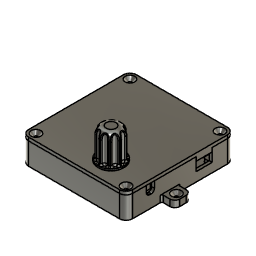
case_esp32_switch_v12 (Autodesk Fusion 360 design; units mm, degrees)
Autodesk Fusion 360 part; units mm, degrees
sketch "Skizze1" plane through (0, 0, 0) normal (0, 0, 1) x (1, 0, 0)
  line L0 (-30, 17.5) -> (30, 17.5)
  line L1 (30, 17.5) -> (30, -17.5)
  line L2 (30, -17.5) -> (-30, -17.5)
  line L3 (-30, -17.5) -> (-30, 17.5)
  line L4 (27.5, -15) -> (-27.5, -15) construction
  line L5 (-27.5, -15) -> (-27.5, 15) construction
  line L6 (-27.5, 15) -> (27.5, 15) construction
  line L7 (27.5, 15) -> (27.5, -15) construction
  line L8 (-22.2, 17.5) -> (-4.2, 17.5)
  line L9 (-4.2, 17.5) -> (-4.2, 22.9)
  line L10 (-4.2, 22.9) -> (-22.2, 22.9)
  line L11 (-22.2, 22.9) -> (-22.2, 17.5)
  line L12 (-30, 1.6) -> (-24, 1.6)
  line L13 (-24, 1.6) -> (-24, -7.6)
  line L14 (-24, -7.6) -> (-30, -7.6)
  line L15 (-30, -7.6) -> (-30, 1.6)
  line L16 (30, 11.5) -> (21, 11.5)
  line L17 (21, 11.5) -> (21, 1.6)
  line L18 (21, 1.6) -> (30, 1.6)
  line L19 (30, 1.6) -> (30, 11.5)
  line L20 (0, 17.5) -> (0, 0) construction
  line L21 (0, 0) -> (-30, 0) construction
  line L22 (30.2, -17.7) -> (-30.2, -17.7)
  line L23 (-30.2, -17.7) -> (-30.2, 17.7)
  line L24 (-30.2, 17.7) -> (30.2, 17.7)
  line L25 (30.2, 17.7) -> (30.2, -17.7)
  line L26 (-32, -41.5) -> (-32, 24.9)
  line L27 (-32, 24.9) -> (32, 24.9)
  line L28 (32, 24.9) -> (32, -41.5)
  line L29 (32, -41.5) -> (-32, -41.5)
  line L30 (-30.2, 17.7) -> (-30.2, 23.1)
  line L31 (-30.2, 23.1) -> (32, 23.1)
  line L32 (-30, 1.6) -> (-32, 1.6)
  line L33 (-30, -7.6) -> (-32, -7.6)
  line L34 (30, 11.5) -> (32, 11.5)
  line L35 (30, 1.6) -> (32, 1.6)
  line L36 (25.2, 17.7) -> (30.2, 17.7)
  line L37 (30.2, 17.7) -> (30.2, 12.7)
  line L38 (30.2, 12.7) -> (25.2, 12.7)
  line L39 (25.2, 12.7) -> (25.2, 17.7)
  line L40 (-30.2, 17.7) -> (-25.2, 17.7)
  line L41 (-25.2, 17.7) -> (-25.2, 12.7)
  line L42 (-25.2, 12.7) -> (-30.2, 12.7)
  line L43 (-30.2, 12.7) -> (-30.2, 17.7)
  line L44 (-30.2, -17.7) -> (-25.2, -17.7)
  line L45 (-25.2, -17.7) -> (-25.2, -12.7)
  line L46 (-25.2, -12.7) -> (-30.2, -12.7)
  line L47 (-30.2, -12.7) -> (-30.2, -17.7)
  line L48 (30.2, -17.7) -> (25.2, -17.7)
  line L49 (25.2, -17.7) -> (25.2, -12.7)
  line L50 (25.2, -12.7) -> (30.2, -12.7)
  line L51 (30.2, -12.7) -> (30.2, -17.7)
  line L52 (30.2, -17.7) -> (30.2, -39.7)
  line L53 (30.2, -39.7) -> (-30.2, -39.7)
  line L54 (-30.2, -39.7) -> (-30.2, -17.7)
  line L55 (-4.3, -19.2) -> (22.2, -19.2)
  line L56 (22.2, -19.2) -> (22.2, -38)
  line L57 (22.2, -38) -> (-4.3, -38)
  line L58 (-4.3, -38) -> (-4.3, -19.2)
  line L59 (22.2, -21.45) -> (-4.3, -21.45) construction
  line L60 (30.2, 17.7) -> (30.2, 23.1)
  line L61 (22.2, -23.3) -> (-4.3, -23.3)
  line L62 (22.2, -36) -> (-4.3, -36)
  line L63 (-30.2, 23.1) -> (-25.2, 23.1)
  line L64 (-25.2, 23.1) -> (-25.2, 18.1)
  line L65 (-25.2, 18.1) -> (-30.2, 18.1)
  line L66 (-30.2, 18.1) -> (-30.2, 23.1)
  line L67 (30.2, 23.1) -> (25.2, 23.1)
  line L68 (25.2, 23.1) -> (25.2, 18.1)
  line L69 (25.2, 18.1) -> (30.2, 18.1)
  line L70 (30.2, 18.1) -> (30.2, 23.1)
  line L71 (30.2, -39.7) -> (25.2, -39.7)
  line L72 (25.2, -39.7) -> (25.2, -34.7)
  line L73 (25.2, -34.7) -> (30.2, -34.7)
  line L74 (30.2, -34.7) -> (30.2, -39.7)
  line L75 (-30.2, -39.7) -> (-25.2, -39.7)
  line L76 (-25.2, -39.7) -> (-25.2, -34.7)
  line L77 (-25.2, -34.7) -> (-30.2, -34.7)
  line L78 (-30.2, -34.7) -> (-30.2, -39.7)
  line L79 (23.4, -39.2) -> (-5.5, -39.2)
  line L80 (-5.5, -39.2) -> (-5.5, -18)
  line L81 (-5.5, -18) -> (23.4, -18)
  line L82 (23.4, -18) -> (23.4, -39.2)
  line L83 (-4.3, -23.3) -> (-5.5, -23.3)
  line L84 (22.2, -23.3) -> (23.4, -23.3)
  line L85 (22.2, -36) -> (23.4, -36)
  line L86 (-4.3, -36) -> (-5.5, -36)
  point P0 (2.7, -21.45)
  point P1 (16.4, -21.45)
  dimension "d1" = 35
  dimension "d2" = 60
  dimension "d3" = 2.5
  dimension "d4" = 18
  dimension "d5" = 7.8
  dimension "d6" = 9.2
  dimension "d7" = 9.9
  dimension "d8" = 5.4
  dimension "d9" = 9.9
  dimension "d10" = 6
  dimension "d11" = 9
  dimension "d12" = 6
  dimension "d13" = -0.2
  dimension "d14" = 2
  dimension "d15" = 1.8
  dimension "d16" = 1.8
  dimension "d17" = 1.8
  dimension "d18" = 5
  dimension "d19" = 5
  dimension "d20" = 5
  dimension "d21" = 5
  dimension "d22" = 22
  dimension "d23" = 1.8
  dimension "d24" = 26.5
  dimension "d25" = 18.8
  dimension "d26" = 8
  dimension "d27" = 2.25
  dimension "d28" = 13.7
  dimension "d29" = 7
  dimension "d30" = 1.5
  dimension "d38" = 4.1
  dimension "d39" = 2
  dimension "d43" = 5
  dimension "d44" = 5
  dimension "d45" = 5
  dimension "d46" = 5
  dimension "d57" = -1.2
  constraint horizontal L0
  constraint vertical L1
  constraint horizontal L2
  constraint vertical L3
  constraint horizontal L8
  constraint vertical L9
  constraint horizontal L10
  constraint vertical L11
  constraint coincident L0 L8.start
  constraint horizontal L12
  constraint vertical L13
  constraint horizontal L14
  constraint vertical L15
  constraint coincident L3 L12.start
  constraint horizontal L16
  constraint vertical L17
  constraint horizontal L18
  constraint vertical L19
  constraint coincident L1 L16.start
  constraint midpoint L0 L20.start
  constraint coincident L20.end L21.start
  constraint midpoint L3 L21.end
  constraint horizontal L21
  constraint vertical L20
  constraint vertical L26
  constraint perpendicular L26 L27
  constraint perpendicular L27 L28
  constraint perpendicular L26 L29
  constraint perpendicular L27 L30
  constraint coincident L28 L31.end
  constraint perpendicular L28 L31
  constraint coincident L26 L32.end
  constraint perpendicular L26 L32
  constraint coincident L26 L33.end
  constraint perpendicular L26 L33
  constraint coincident L28 L34.end
  constraint perpendicular L28 L34
  constraint coincident L28 L35.end
  constraint perpendicular L28 L35
  constraint horizontal L36
  constraint vertical L37
  constraint horizontal L38
  constraint vertical L39
  constraint coincident L25 L37.end
  constraint coincident L24 L36.start
  constraint horizontal L40
  constraint vertical L41
  constraint horizontal L42
  constraint vertical L43
  constraint horizontal L44
  constraint vertical L45
  constraint horizontal L46
  constraint vertical L47
  constraint horizontal L48
  constraint vertical L49
  constraint horizontal L50
  constraint vertical L51
  constraint collinear L39 L49
  constraint collinear L46 L50
  constraint collinear L41 L45
  constraint collinear L38 L42
  constraint perpendicular L48 L52
  constraint perpendicular L25 L53
  constraint perpendicular L53 L54
  constraint horizontal L55
  constraint vertical L56
  constraint horizontal L57
  constraint vertical L58
  constraint coincident L56 L59.start
  constraint coincident L58 L59.end
  constraint perpendicular L58 L59
  constraint coincident L59 P0
  constraint coincident L59 P1
  constraint perpendicular L31 L60
  constraint coincident L56 L61.start
  constraint coincident L58 L61.end
  constraint perpendicular L58 L61
  constraint coincident L56 L62.start
  constraint coincident L58 L62.end
  constraint perpendicular L58 L62
  constraint horizontal L63
  constraint vertical L64
  constraint horizontal L65
  constraint vertical L66
  constraint horizontal L67
  constraint vertical L68
  constraint horizontal L69
  constraint vertical L70
  constraint horizontal L71
  constraint vertical L72
  constraint horizontal L73
  constraint vertical L74
  constraint horizontal L75
  constraint vertical L76
  constraint horizontal L77
  constraint vertical L78
  constraint collinear L64 L76
  constraint collinear L73 L77
  constraint collinear L68 L72
  constraint collinear L65 L69
  constraint coincident L80 L83.end
  constraint perpendicular L80 L83
  constraint coincident L82 L84.end
  constraint perpendicular L82 L84
  constraint coincident L82 L85.end
  constraint perpendicular L82 L85
  constraint coincident L80 L86.end
  constraint perpendicular L80 L86
  measures "d1" distance of L0 L2
  measures "d2" distance of L1 L3
  measures "d4" distance of L9.end L10.end
  measures "d5" distance of L3 L11
  measures "d6" distance of L12.end L13.end
  measures "d7" distance of L2 L14
  measures "d8" distance of L8.start L10.end
  measures "d9" distance of L16.end L17.end
  measures "d10" distance of L0 L16
  measures "d11" distance of L17.end L18.end
  measures "d12" distance of L13.end L14.end
  measures "d14" distance of L10 L27
  measures "d15" distance of L26 L30
  measures "d16" distance of L27 L31
  measures "d17" distance of L25 L28
  measures "d18" distance of L37 L39
  measures "d19" distance of L24 L38
  measures "d20" distance of L45.end L46.end
  measures "d21" distance of L44.end L45.end
  measures "d22" distance of L22 L53
  measures "d23" distance of L29 L53
  measures "d24" distance of L56.end L57.end
  measures "d25" distance of L55.end L56.end
  measures "d26" distance of L52 L56
  measures "d27" distance of L55 L59
  measures "d28" distance of P0 P1
  measures "d29" distance of L58 P0
  measures "d30" distance of L22 L55
  measures "d38" distance of L55 L61
  measures "d39" distance of L57 L62
  measures "d43" distance of L64.end L65.end
  measures "d44" distance of L63.end L64.end
  measures "d45" distance of L75.end L76.end
  measures "d46" distance of L60 L68
extrude "Extrusion1" add sketch "Skizze1" against normal blind 2 contours L0 L8 L9 L11 L24 | L0 L1 L2 L3 L8 L12 L13 L14 L16 L17 L18 L38 L39 L41 L42 L45 L46 L49 L50 | L0 L11 L24 L41 | L0 L9 L24 L39 | L0 L3 L41 L42 | L0 L3 L23 L24 L40 L41 L42 L43 | L9 L10 L11 L24 L30 L31 L36 L40 L60 L64 L65 L68 L69 | L9 L10 L11 L24 | L0 L1 L24 L25 L36 L37 L38 L39 | L0 L1 L38 L39 | L3 L23 L32 L42 | L23 L26 L27 L28 L30 L31 L32 L43 L63 L66 L67 | L1 L25 L34 L38 | L25 L28 L31 L34 L37 L60 L70 | L3 L12 L13 L14 L15 | L3 L15 L23 L32 L33 | L30 L31 L63 L64 L65 L66 | L1 L19 L25 L34 L35 | L1 L16 L17 L18 L19 | L31 L60 L67 L68 L69 L70 | L3 L23 L33 L46 | L23 L26 L32 L33 | L1 L25 L35 L50 | L25 L28 L34 L35 | L2 L3 L45 L46 | L2 L3 L22 L23 L44 L45 L46 L47 | L23 L25 L26 L28 L29 L33 L35 L47 L51 L52 L53 L54 L71 L74 L75 L78 | L1 L2 L22 L25 L48 L49 L50 L51 | L1 L2 L49 L50 | L2 L22 L45 L49 | L22 L44 L48 L52 L53 L54 L72 L73 L76 L77 | L53 L54 L75 L76 L77 L78 | L52 L53 L71 L72 L73 L74 | L55 L56 L58 L80 L81 L82 L83 L84 | L55 L56 L58 L61 | L56 L58 L61 L62 | L58 L80 L83 L86 | L56 L82 L84 L85 | L56 L57 L58 L62 | L56 L57 L58 L79 L80 L82 L85 L86 makes body 1
extrude "Extrusion2" add sketch "Skizze1" along normal blind 2 contours L0 L3 L41 L42 | L0 L3 L23 L24 L40 L41 L42 L43 | L0 L1 L24 L25 L36 L37 L38 L39 | L0 L1 L38 L39 | L23 L26 L27 L28 L30 L31 L32 L43 L63 L66 L67 | L25 L28 L31 L34 L37 L60 L70 | L23 L26 L32 L33 | L25 L28 L34 L35 | L2 L3 L45 L46 | L2 L3 L22 L23 L44 L45 L46 L47 | L23 L25 L26 L28 L29 L33 L35 L47 L51 L52 L53 L54 L71 L74 L75 L78 | L1 L2 L22 L25 L48 L49 L50 L51 | L1 L2 L49 L50 | L55 L56 L58 L61 | L56 L57 L58 L62 bodies 1
extrude "Extrusion3" add sketch "Skizze1" along normal blind 1.55 from surface at 2 contours L23 L26 L27 L28 L30 L31 L32 L43 L63 L66 L67 | L25 L28 L31 L34 L37 L60 L70 | L23 L26 L32 L33 | L25 L28 L34 L35 | L23 L25 L26 L28 L29 L33 L35 L47 L51 L52 L53 L54 L71 L74 L75 L78 bodies 1
extrude "Extrusion4" add sketch "Skizze1" along normal blind 7.95 from surface at 3.55 contours L23 L26 L27 L28 L30 L31 L32 L43 L63 L66 L67 | L25 L28 L31 L34 L37 L60 L70 | L23 L25 L26 L28 L29 L33 L35 L47 L51 L52 L53 L54 L71 L74 L75 L78 bodies 1
extrude "Extrusion5" add sketch "Skizze1" along normal up to surface (10.5 mm away) contours L30 L31 L63 L64 L65 L66 | L31 L60 L67 L68 L69 L70 | L53 L54 L75 L76 L77 L78 | L52 L53 L71 L72 L73 L74 bodies 1
fillet "Abrundung1" radius 4 8 edges at (-32, -41.5, 4.75) (32, -41.5, 4.75) (-32, 24.9, 4.75) (32, 24.9, 4.75) (30.2, 23.1, 11) (-30.2, 23.1, 11) (-30.2, -39.7, 11) (30.2, -39.7, 11) on bodies 1
sketch "Skizze2" plane through (0, 0, 2) normal (0, 0, 1) x (-1, 0, 0)
  line L0 (-22.2, 23.3) -> (-22.2, 19.2)
  line L1 (-22.2, 19.2) -> (4.3, 19.2)
  line L2 (4.3, 19.2) -> (4.3, 23.3)
  line L3 (4.3, 23.3) -> (-22.2, 23.3)
  point P0 (-2.7, 21.45)
  point P1 (-2.7, 21.45)
  point P2 (-16.4, 21.45)
  point P3 (-16.4, 21.45)
  constraint coincident P1 P0
  constraint coincident P3 P2
sketch "Skizze3" plane through (0, 0, 2) normal (0, 0, 1) x (-1, 0, 0)
  line L0 (30.2, -17.7) -> (30.2, -12.7)
  line L1 (30.2, -12.7) -> (25.2, -12.7)
  line L2 (25.2, -12.7) -> (25.2, -17.7)
  line L3 (25.2, -17.7) -> (30.2, -17.7)
  point P0 (27.5, -15)
  point P1 (27.5, -15)
  point P2 (27.5, 15)
  point P3 (27.5, 15)
  point P4 (-27.5, 15)
  point P5 (-27.5, 15)
  point P6 (-27.5, -15)
  point P7 (-27.5, -15)
  constraint coincident P1 P0
  constraint coincident P3 P2
  constraint coincident P5 P4
  constraint coincident P7 P6
hole "Bohrung1" at (-27.5, -15, 2) at (-27.5, 15, 2) at (27.5, 15, 2) at (27.5, -15, 2) direction (0, 0, -1) diameter 1.4 depth 3 tip angle 180 bodies 1
hole "Bohrung2" at (2.7, -21.45, 2) at (16.4, -21.45, 2) direction (0, 0, -1) diameter 1.4 depth 3 tip angle 180 bodies 1
sketch "Skizze4" plane through (0, 0, 10.5) normal (0, 0, 1) x (-1, 0, 0)
  arc A0 (30.2, 35.7) -> (26.2, 39.7) centre (26.2, 35.7) ccw
  line L0 (26.2, 39.7) -> (25.2, 39.7)
  line L1 (25.2, 39.7) -> (25.2, 34.7)
  line L2 (25.2, 34.7) -> (30.2, 34.7)
  line L3 (30.2, 34.7) -> (30.2, 35.7)
extrude "Extrusion6" add sketch "Skizze1" along normal up to surface (4 mm away) contours L55 L56 L58 L80 L81 L82 L83 L84 | L56 L57 L58 L79 L80 L82 L85 L86 bodies 1
sketch "Skizze5" plane through (0, 0, 10.5) normal (0, 0, 1) x (-1, 0, 0)
  point P0 (27.7, 37.2)
  point P1 (27.7, -20.6)
  point P2 (-27.7, -20.6)
  point P3 (-27.7, 37.2)
hole "Bohrung3" at (-27.7, 20.6, 10.5) at (27.7, 20.6, 10.5) at (27.7, -37.2, 10.5) at (-27.7, -37.2, 10.5) direction (0, 0, -1) diameter 1.4 depth 8 tip angle 180 bodies 1
fillet "Abrundung2" radius 1.5 2 edges at (-31.1, 1.6, 3.55) (-31.1, -7.6, 3.55) on bodies 1
fillet "Abrundung3" radius 2 4 edges at (-25.2, -34.7, 5.25) (-25.2, 18.1, 5.25) (25.2, 18.1, 5.25) (25.2, -34.7, 5.25) on bodies 1
fillet "Abrundung4" radius 1 14 edges at (-25.2, -17.7, 1) (-25.2, -12.7, 1) (-25.2, 12.7, 1) (-25.2, 17.7, 1) (25.2, 12.7, 1) (25.2, 17.7, 1) (25.2, -12.7, 1) (25.2, -17.7, 1) (30.2, -17.7, 1) (30.2, -12.7, 1) (30.2, 12.7, 1) (-30.2, 12.7, 1) (-30.2, -17.7, 1) (-30.2, -12.7, 1) on bodies 1
sketch "Skizze6" plane through (0, 0, -2) normal (0, 0, -1) x (1, 0, 0)
  arc A0 (28, -24.9) -> (32, -20.9) centre (28, -20.9) ccw
  line L0 (32, -20.9) -> (32, 37.5)
  arc A1 (32, 37.5) -> (28, 41.5) centre (28, 37.5) ccw
  line L1 (28, 41.5) -> (-28, 41.5)
  arc A2 (-28, 41.5) -> (-32, 37.5) centre (-28, 37.5) ccw
  line L2 (-32, 37.5) -> (-32, -20.9)
  arc A3 (-32, -20.9) -> (-28, -24.9) centre (-28, -20.9) ccw
  line L3 (-28, -24.9) -> (28, -24.9)
  line L4 (-32, 9.5) -> (-40, 9.5)
  line L5 (-40, 9.5) -> (-40, 19.5)
  line L6 (-40, 19.5) -> (-32, 19.5)
  line L7 (-32, 19.5) -> (-32, 9.5)
  line L8 (32, 9.5) -> (40, 9.5)
  line L9 (40, 9.5) -> (40, 19.5)
  line L10 (40, 19.5) -> (32, 19.5)
  line L11 (32, 19.5) -> (32, 9.5)
  line L12 (32, 41.5) -> (-32, 41.5)
  dimension "d69" = 10
  dimension "d70" = 8
  dimension "d71" = 8
  dimension "d72" = 22
  constraint horizontal L4
  constraint vertical L5
  constraint horizontal L6
  constraint vertical L7
  constraint coincident L2 L4.start
  constraint horizontal L8
  constraint vertical L9
  constraint horizontal L10
  constraint vertical L11
  constraint coincident L0 L8.start
  constraint collinear L6 L10
  constraint collinear L4 L8
  measures "d69" distance of L4.end L5.end
  measures "d70" distance of L4.start L4.end
  measures "d71" distance of L8.start L8.end
  measures "d72" distance of L6 L12
extrude "Extrusion7" add sketch "Skizze6" against normal blind 4 contours L0 L8 L9 L10 L11 | L2 L4 L5 L6 L7 bodies 1
fillet "Abrundung5" radius 3 4 edges at (40, -9.5, 0) (40, -19.5, 0) (-40, -19.5, 0) (-40, -9.5, 0) on bodies 1
fillet "Abrundung6" radius 1 4 edges at (32, -19.5, 0) (32, -9.5, 0) (-32, -9.5, 0) (-32, -19.5, 0) on bodies 1
sketch "Skizze7" plane through (0, 0, 2) normal (0, 0, 1) x (-1, 0, 0)
  arc A0 (-37, 19.5) -> (-40, 16.5) centre (-37, 16.5) ccw
  line L0 (-40, 16.5) -> (-40, 12.5)
  arc A1 (-40, 12.5) -> (-37, 9.5) centre (-37, 12.5) ccw
  line L1 (-37, 9.5) -> (-33, 9.5)
  arc A2 (-32, 8.5) -> (-33, 9.5) centre (-33, 8.5) ccw
  line L2 (-32, 8.5) -> (-32, 20.5)
  arc A3 (-33, 19.5) -> (-32, 20.5) centre (-33, 20.5) ccw
  line L3 (-33, 19.5) -> (-37, 19.5)
  line L4 (40, 12.5) -> (40, 16.5)
  line L5 (-40, 14.5) -> (40, 14.5) construction
  line L6 (-40, 9.5) -> (-40, 19.5)
  point P0 (-36, 14.5)
  point P1 (36, 14.5)
  point P2 (40, 19.5)
  dimension "d84" = 4
  dimension "d85" = 4
  constraint midpoint L0 L5.start
  constraint midpoint L4 L5.end
  constraint coincident P1 L5
  constraint coincident P0 L5
  measures "d84" distance of P0 L6
  measures "d85" horizontal distance of P1 P2
hole "Bohrung4" at (-36, -14.5, 2) at (36, -14.5, 2) direction (0, 0, -1) diameter 2 depth 8 tip angle 180 countersink diameter 6 countersink angle 90 bodies 1
sketch "Skizze1 (2)" plane through (0, 0, 11.5) normal (0, 0, 1) x (-1, 0, 0) in component "top"
  arc A0 (-32, -20.9) -> (-28, -24.9) centre (-28, -20.9) ccw
  line L0 (-28, -24.9) -> (28, -24.9)
  arc A1 (28, -24.9) -> (32, -20.9) centre (28, -20.9) ccw
  line L1 (32, -20.9) -> (32, -1.6)
  line L2 (32, -1.6) -> (30.2, -1.6)
  line L3 (30.2, -1.6) -> (30.2, -19.1)
  arc A2 (26.2, -23.1) -> (30.2, -19.1) centre (26.2, -19.1) ccw
  line L4 (26.2, -23.1) -> (-26.2, -23.1)
  arc A3 (-30.2, -19.1) -> (-26.2, -23.1) centre (-26.2, -19.1) ccw
  line L5 (-30.2, -19.1) -> (-30.2, -11.5)
  line L6 (-30.2, -11.5) -> (-32, -11.5)
  line L7 (-32, -11.5) -> (-32, -20.9)
  arc A4 (-28, 41.5) -> (-32, 37.5) centre (-28, 37.5) ccw
  line L8 (-32, 37.5) -> (-32, -1.6)
  line L9 (-32, -1.6) -> (-30.2, -1.6)
  line L10 (-30.2, -1.6) -> (-30.2, 35.7)
  arc A5 (-26.2, 39.7) -> (-30.2, 35.7) centre (-26.2, 35.7) ccw
  line L11 (-26.2, 39.7) -> (26.2, 39.7)
  arc A6 (30.2, 35.7) -> (26.2, 39.7) centre (26.2, 35.7) ccw
  line L12 (30.2, 35.7) -> (30.2, 7.6)
  line L13 (30.2, 7.6) -> (32, 7.6)
  line L14 (32, 7.6) -> (32, 37.5)
  arc A7 (32, 37.5) -> (28, 41.5) centre (28, 37.5) ccw
  line L15 (28, 41.5) -> (-28, 41.5)
  circle A8 centre (27.7, -20.6) radius 0.7
  circle A9 centre (-27.7, -20.6) radius 0.7
  circle A10 centre (-27.7, 37.2) radius 0.7
  circle A11 centre (27.7, 37.2) radius 0.7
  circle A12 centre (27.5, 15) radius 0.7
  circle A13 centre (-11.2, 29.9) radius 3.75
  line L16 (32, -1.6) -> (32, 7.6)
  line L17 (30.2, -1.6) -> (30.2, 7.6)
  line L18 (-30.2, -11.5) -> (-30.2, -1.6)
  line L19 (-32, -11.5) -> (-32, -1.6)
  arc A14 (26.2, -23) -> (30.1, -19.1) centre (26.2, -19.1) ccw
  line L20 (30.1, -1.5) -> (30.1, -19.1)
  line L21 (32.1, -1.5) -> (30.1, -1.5)
  line L22 (32.1, -20.9) -> (32.1, -1.5)
  arc A15 (28, -25) -> (32.1, -20.9) centre (28, -20.9) ccw
  line L23 (-28, -25) -> (28, -25)
  arc A16 (-32.1, -20.9) -> (-28, -25) centre (-28, -20.9) ccw
  line L24 (-32.1, -11.4) -> (-32.1, -20.9)
  line L25 (-30.1, -11.4) -> (-32.1, -11.4)
  line L26 (-30.1, -19.1) -> (-30.1, -11.4)
  arc A17 (-30.1, -19.1) -> (-26.2, -23) centre (-26.2, -19.1) ccw
  line L27 (26.2, -23) -> (-26.2, -23)
  line L28 (32.1, 7.5) -> (32.1, 37.5)
  arc A18 (32.1, 37.5) -> (28, 41.6) centre (28, 37.5) ccw
  line L29 (28, 41.6) -> (-28, 41.6)
  arc A19 (-28, 41.6) -> (-32.1, 37.5) centre (-28, 37.5) ccw
  line L30 (-32.1, 37.5) -> (-32.1, -1.7)
  line L31 (-32.1, -1.7) -> (-30.1, -1.7)
  line L32 (-30.1, -1.7) -> (-30.1, 35.7)
  arc A20 (-26.2, 39.6) -> (-30.1, 35.7) centre (-26.2, 35.7) ccw
  line L33 (-26.2, 39.6) -> (26.2, 39.6)
  arc A21 (30.1, 35.7) -> (26.2, 39.6) centre (26.2, 35.7) ccw
  line L34 (30.1, 35.7) -> (30.1, 7.5)
  line L35 (30.1, 7.5) -> (32.1, 7.5)
  line L36 (30.1, -1.5) -> (30.1, 7.5)
  line L37 (-30.1, -11.4) -> (-30.1, -1.7)
  line L38 (32, 7.5) -> (27, 7.5)
  line L39 (27, 7.5) -> (27, -1.5)
  line L40 (27, -1.5) -> (32, -1.5)
  line L41 (32, -1.5) -> (32, 7.5)
  line L42 (-32, -1.7) -> (-27, -1.7)
  line L43 (-27, -1.7) -> (-27, -11.4)
  line L44 (-27, -11.4) -> (-32, -11.4)
  line L45 (-32, -11.4) -> (-32, -1.7)
  dimension "d86" = 7.5
  dimension "d87" = 0.1
  dimension "d88" = 0.1
  dimension "d91" = 11.6
  dimension "d92" = 20.8
  dimension "d144" = 5
  dimension "d145" = 5
  constraint coincident L1.end L2.start
  constraint coincident L13.end L14.start
  constraint coincident L2.end L3.start
  constraint coincident L12.end L13.start
  constraint coincident L5.end L6.start
  constraint coincident L9.end L10.start
  constraint coincident L6.end L7.start
  constraint coincident L8.end L9.start
  constraint perpendicular L35 L36
  constraint perpendicular L31 L37
  constraint horizontal L38
  constraint vertical L39
  constraint horizontal L40
  constraint vertical L41
  constraint coincident L35 L38.start
  constraint coincident L16 L38.start
  constraint coincident L21 L40.end
  constraint horizontal L42
  constraint vertical L43
  constraint horizontal L44
  constraint vertical L45
  constraint coincident L19 L42.start
  constraint coincident L31 L42.start
  constraint coincident L25 L44.end
  measures "d86" diameter of A13
  measures "d91" distance of L15 A13.centre
  measures "d92" distance of L8 A13.centre
  measures "d144" distance of L38.start L38.end
  measures "d145" distance of L42.start L42.end
extrude "Extrusion1'" add sketch "Skizze1 (2)" along normal blind 2 separate body contours A0 L0 A1 L1 L2 L3 A2 L4 A3 L5 L6 L7 | L6 L18 L19 L25 L44 | L3 A2 L4 A3 L5 L17 L18 A14 L20 L21 L25 L26 A17 L27 L40 L44 | L18 L19 L25 L31 L42 L44 L45 | L18 L25 L31 L37 L42 L44 | L9 L18 L19 L31 L42 | L2 L16 L17 L21 L40 | L10 A5 L11 A6 L12 L17 L18 L31 L32 A20 L33 A21 L34 L35 L38 L42 | A14 L20 L26 A17 L27 L32 A20 L33 A21 L34 L38 L39 L40 L42 L43 L44 | L37 L42 L43 L44 | A4 L8 L9 L10 A5 L11 A6 L12 L13 L14 A7 L15 | L16 L17 L21 L35 L38 L40 L41 | L17 L21 L35 L36 L38 L40 | L13 L16 L17 L35 L38 | L36 L38 L39 L40 | A8 | A9 | A10 | A11 | A12 makes body 2 in component "top"
extrude "Extrusion2'" add sketch "Skizze1 (2)" against normal blind 0.85 contours A14 L20 L26 A17 L27 L32 A20 L33 A21 L34 L38 L39 L40 L42 L43 L44 | L37 L42 L43 L44 | L36 L38 L39 L40 | A8 | A9 | A10 | A12 bodies 2 in component "top"
extrude "Extrusion3'" add sketch "Skizze1 (2)" against normal blind 2.4 contours L18 L19 L25 L31 L42 L44 L45 bodies 2 in component "top"
extrude "Extrusion4'" add sketch "Skizze1 (2)" against normal blind 4.4 contours L16 L17 L21 L35 L38 L40 L41 bodies 2 in component "top"
sketch "Skizze2 (2)" plane through (0, 0, 13.5) normal (0, 0, 1) x (-1, 0, 0) in component "top"
  circle A0 centre (-11.2, 29.9) radius 3.75
  arc A1 (-32, -20.9) -> (-28, -24.9) centre (-28, -20.9) ccw
  line L0 (-28, -24.9) -> (28, -24.9)
  arc A2 (28, -24.9) -> (32, -20.9) centre (28, -20.9) ccw
  line L1 (32, -20.9) -> (32, 37.5)
  arc A3 (32, 37.5) -> (28, 41.5) centre (28, 37.5) ccw
  line L2 (28, 41.5) -> (-28, 41.5)
  arc A4 (-28, 41.5) -> (-32, 37.5) centre (-28, 37.5) ccw
  line L3 (-32, 37.5) -> (-32, -20.9)
  point P0 (-27.7, 37.2)
  point P1 (-27.7, -20.6)
  point P2 (27.7, -20.6)
  point P3 (27.7, 37.2)
hole "Bohrung5" at (28, -37.5, 13.5) at (27.7, 20.6, 13.5) at (-27.7, 20.6, 13.5) at (-27.7, -37.2, 13.5) direction (0, 0, -1) diameter 2 depth 8 tip angle 180 countersink diameter 6 countersink angle 90 bodies 1
hole "Bohrung1'" at (28, -37.5, 13.5) at (27.7, 20.6, 13.5) at (-27.7, 20.6, 13.5) at (-27.7, -37.2, 13.5) direction (0, 0, -1) diameter 2 depth 8 tip angle 180 countersink diameter 6 countersink angle 90 bodies 2 in component "top"
sketch "Skizze1 (3)" plane through (0, 0, 13.5) normal (0, 0, 1) x (-1, 0, 0) in component "knob"
  circle A0 centre (-11.2, 29.9) radius 7
  circle A1 centre (-11.2, 29.9) radius 3
  line L0 (-13.8263, 31.35) -> (-8.5737, 31.35)
  line L1 (-11.2, 31.35) -> (-11.2, 26.9)
  point P0 (-11.2, 29.9)
  dimension "d111" = 14
  dimension "d112" = 6
  dimension "d113" = 4.45
  constraint coincident P0 A0.centre
  constraint coincident A1 L0.start
  constraint coincident A1 L0.end
  constraint horizontal L0
  constraint midpoint L0 L1.start
  constraint coincident A1 L1.end
  constraint perpendicular L0 L1
  measures "d111" diameter of A0
  measures "d112" diameter of A1
  measures "d113" distance of L1.start L1.end
extrude "Extrusion1''" add sketch "Skizze1 (3)" along normal blind 20 separate body makes body 3 in component "knob"
sketch "Skizze2 (3)" plane through (0, 0, 33.5) normal (0, 0, 1) x (-1, 0, 0) in component "knob"
  circle A0 centre (-11.2, 29.9) radius 3
  circle A1 centre (-11.2, 29.9) radius 7
  line L0 (-13.8263, 31.35) -> (-8.5737, 31.35)
extrude "Extrusion2''" add sketch "Skizze2 (3)" against normal blind 2 contours A0 L0 picked at (-11.876, 28.1713) bodies 3 in component "knob"
extrude "Extrusion3''" add sketch "Skizze2 (3)" against normal blind 12 contours A0 L0 picked at (-11.129, 31.8641) bodies 3 in component "knob"
extrude "Extrusion4''" cut sketch "Skizze1 (3)" along normal blind 1 bodies 3 in component "knob"
sketch "Skizze3 (2)" plane through (0, 0, 14.5) normal (0, 0, -1) x (1, 0, 0) in component "knob"
  circle A0 centre (11.2, 29.9) radius 3
  circle A1 centre (11.2, 29.9) radius 7
  circle A2 centre (11.2, 29.9) radius 8
  dimension "d122" = 16
  constraint concentric A0 A2
  measures "d122" diameter of A2
extrude "Extrusion5'" add sketch "Skizze3 (2)" against normal blind 1.5 contours A2 bodies 3 in component "knob"
sketch "Skizze4 (2)" plane through (0, 0, 33.5) normal (0, 0, 1) x (-1, 0, 0) in component "knob"
  circle A0 centre (-11.2, 29.9) radius 7
  circle A1 centre (-11.2, 22.9) radius 1.5
  circle A2 centre (-11.2, 36.9) radius 1
  line L0 (-11.2, 29.9) -> (-11.2, 36.9) construction
  line L1 (-11.2, 29.9) -> (-11.2, 22.9) construction
  dimension "d125" = 3
  dimension "d134" = 2
  constraint coincident A0 A1.centre
  constraint coincident A0 A2.centre
  constraint coincident A0.centre L0.start
  constraint coincident A2.centre L0.end
  constraint vertical L0
  constraint coincident A1.centre L1.end
  constraint parallel L0 L1
  measures "d125" diameter of A1
  measures "d134" diameter of A2
fillet "Abrundung4'" radius 4 1 edges at (17.7263, -27.3687, 33.5) on bodies 3 in component "knob"
extrude "Extrusion6'" cut sketch "Skizze4 (2)" against normal up to surface (17.5 mm away) contours A0 A1 picked at (-11.2, 23.4119) bodies 3 in component "knob"
pattern_circular "C-Anordnung1" count 9 over 360 about axis through (11.2, -29.9, 13.5) along (0, 0, 1) of "Extrusion6'" in component "knob"
fillet "Abrundung1'" radius 0.6 28 edges at (6.0227, -34.6112, 22.75) (6.3293, -32.4888, 32.6097) (4.5313, -32.0281, 22.75) (4.2056, -30.1811, 22.75) (5.8048, -28.7522, 32.6097) (4.7236, -27.2437, 22.75) (5.6613, -25.6194, 22.75) (7.8051, -25.5525, 32.6096) (7.9462, -23.7022, 22.75) (9.7086, -23.0607, 22.75) (11.404, -24.3861, 32.6082) (12.6914, -23.0607, 22.75) (17.6764, -27.2437, 22.75) (16.6624, -29.1333, 32.6097) (18.1944, -30.1811, 22.75) (3.7414, -27.0071, 14.5) (17.8687, -32.0281, 22.75) (15.8773, -32.8237, 32.6097) (16.3773, -34.6112, 22.75) (16.7387, -25.6194, 22.75) (14.892, -25.8017, 32.6096) (14.4538, -23.7022, 22.75) (7.4594, -35.8167, 22.75) (9.1344, -35.0143, 32.6099) (10.2623, -36.8369, 22.75) (12.1377, -36.8369, 22.75) (12.9051, -35.1455, 32.6099) (14.9406, -35.8167, 22.75) on bodies 3 in component "knob"
chamfer "Fase1" distance 1 angle 45 36 edges at (15.9631, -32.65, 16) (17.7974, -31.7922, 16) (18.0937, -31.1155, 16) (18.0467, -30.3784, 16) (16.6164, -28.9449, 16) (17.4701, -27.1088, 16) (17.2622, -26.4, 16) (16.7523, -25.8655, 16) (14.7353, -25.6868, 16) (14.209, -23.7314, 16) (13.5941, -23.3222, 16) (12.86, -23.2404, 16) (11.2, -24.4, 16) (9.54, -23.2404, 16) (8.8059, -23.3222, 16) (8.191, -23.7314, 16) (7.6647, -25.6868, 16) (5.6477, -25.8655, 16) (5.1378, -26.4, 16) (4.9299, -27.1088, 16) (5.7836, -28.9449, 16) (4.3533, -30.3784, 16) (4.3063, -31.1155, 16) (4.6026, -31.7922, 16) (6.4369, -32.65, 16) (6.2627, -34.6674, 16) (6.7005, -35.2623, 16) (7.3624, -35.5902, 16) (9.3189, -35.0683, 16) (10.4822, -36.7257, 16) (11.2, -36.9, 16) (11.9178, -36.7257, 16) (13.0811, -35.0683, 16) (15.0376, -35.5902, 16) (15.6995, -35.2623, 16) (16.1373, -34.6674, 16) on bodies 3 in component "knob"
extrude "Extrusion5''" add sketch "Skizze1 (2)" against normal up to surface (2.4 mm away) contours L18 L25 L31 L37 L42 L44 | L37 L42 L43 L44 bodies 2 in component "top"
extrude "Extrusion6''" add sketch "Skizze1 (2)" against normal up to surface (4.4 mm away) contours L17 L21 L35 L36 L38 L40 | L36 L38 L39 L40 bodies 2 in component "top"
sketch "Skizze8" plane through (32, 0, 0) normal (1, 0, 0) x (0, 1, 0)
  line L0 (-8.5, 2) -> (-8.5, -2)
  line L1 (-8.5, -2) -> (20.9, -2)
  line L2 (20.9, -2) -> (20.9, 11.5)
  line L3 (20.9, 11.5) -> (11.5, 11.5)
  line L4 (11.5, 11.5) -> (11.5, 3.55)
  line L5 (11.5, 3.55) -> (1.6, 3.55)
  line L6 (1.6, 3.55) -> (1.6, 11.5)
  line L7 (1.6, 11.5) -> (-37.5, 11.5)
  line L8 (-37.5, 11.5) -> (-37.5, -2)
  line L9 (-37.5, -2) -> (-20.5, -2)
  line L10 (-20.5, -2) -> (-20.5, 2)
  line L11 (-20.5, 2) -> (-8.5, 2)
  line L12 (-29, 11.5) -> (-24, 11.5)
  line L13 (-24, 11.5) -> (-24, 5.5)
  line L14 (-24, 5.5) -> (-29, 5.5)
  line L15 (-29, 5.5) -> (-29, 11.5)
  dimension "d150" = 5
  dimension "d151" = 6
  constraint horizontal L12
  constraint vertical L13
  constraint horizontal L14
  constraint vertical L15
  constraint coincident L7 L12.start
  measures "d150" distance of L13.end L14.end
  measures "d151" distance of L12.start L14.end
extrude "Extrusion8" cut sketch "Skizze8" against normal up to surface (1.8 mm away) contours L7 L12 L13 L14 L15 bodies 1
fillet "Abrundung7" radius 2 2 edges at (31.1, -24, 5.5) (31.1, -29, 5.5) on bodies 1
component "top" placed x (1, 0, 0) y (0, 1, 0) z (0, 0, 1) at (0, 0, 0)
component "knob" placed x (1, 0, 0) y (0, 1, 0) z (0, 0, 1) at (0, 0, 0)
equation "d16 = d15"
equation "d17 = d15"
equation "d20 = d18"
equation "d21 = d18"
equation "d23 = d15"
equation "d41 = 5.2 mm + 3 mm - 0.25 mm"
equation "d91 = 15 mm - ( 6.8 / 2 ) * 1 mm"
equation "d92 = 24.2 mm - ( 6.8 / 2 ) * 1 mm"
